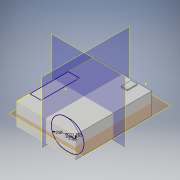
# Autodesk Inventor part: TAZ 6 Convex Model
Saved by Autodesk Inventor 2019 (Build 230136000, 136)
## iProperties
Created: 2021-02-10
Part Number: TAZ 6 Convex Model
Material: Generic
Document SubType Name: Modeling
Designer: Eric
Density: 1 g/cm^3
Appearance: Default
Author: Eric
Autodesk Inventor part; units mm, degrees
ref_plane "YZ Plane" through (0, 0, 0) normal (1, 0, 0) x (0, 1, 0)
ref_plane "XZ Plane" through (0, 0, 0) normal (0, 1, 0) x (-1, 0, 0)
ref_plane "XY Plane" through (0, 0, 0) normal (0, 0, 1) x (1, 0, 0)
ref_plane "Work Plane1" through (-416.1869, -470.7505, 28.2071) normal (0, 0, -1) x (0, 1, 0)
sketch "Sketch1" plane through (-416.1869, -470.7505, 28.2071) normal (0, 0, -1) x (0, 1, 0)
  line L0 (-5.675, 491.5) -> (-5.675, 423.5) construction
  line L1 (170.675, 423.5) -> (170.675, 491.5) construction
  line L2 (166, -7.5) -> (160.638, -7.5) construction
  line L3 (154.362, -7.5) -> (149, -7.5) construction
  line L4 (16, -7.5) -> (10.638, -7.5) construction
  line L5 (4.362, -7.5) -> (-1, -7.5) construction
  line L6 (94.0505, 496.5) -> (100.0959, 496.5) construction
  line L7 (101.0959, 496.5) -> (107.1414, 496.5) construction
  line L8 (108.1414, 496.5) -> (114.1868, 496.5) construction
  line L9 (-13.9999, 496.5) -> (170.675, 496.5)
  line L10 (170.675, 496.5) -> (170.675, -7.5)
  line L11 (170.675, -7.5) -> (-13.9999, -7.5)
  line L12 (-13.9999, -7.5) -> (-13.9999, 496.5)
  line L13 (-13.69, 71.5) -> (-13.69, 253.5) construction
  line L14 (-13.9999, 266.9308) -> (-13.9999, 290.6308) construction
  point P0 (470.7505, 416.1869)
  constraints: 12 end point, 4 collinear, 2 vertical, 4 other
ref_plane "Work Plane2" through (60.3131, -476.4255, 684.8371) normal (0, 0, 1) x (1, 0, 0)
extrude "Extrusion1" add sketch "Sketch1" against normal up to surface (656.63 mm away)
sketch "Sketch2" plane through (-423.6869, -300.0755, 28.2071) normal (0, 1, 0) x (1, 0, 0)
  line L0 (397.25, -16.28) -> (344.1479, -16.28)
  line L1 (344.1479, -16.28) -> (344.1479, -101.13)
  line L2 (344.1479, -101.13) -> (397.25, -101.13)
  line L3 (397.25, -101.13) -> (397.25, -16.28)
  line L4 (344.1479, -35.88) -> (344.1479, -16.38) projected
  arc A0 (397.2117, -88.1724) -> (397.052, -86.959) centre (385.25, -89.13) ccw projected
  line L5 (343.1, -16.28) -> (368.3, -16.28) projected
  point P0 (423.6869, 28.2071)
  constraints: 8 end point, 2 collinear, 2 horizontal, 2 tangent, 2 vertical
ref_plane "Work Plane3" through (-49.4369, -292.7505, 106.3371) normal (0, 1, 0) x (0, 0, 1)
extrude "Extrusion2" add sketch "Sketch2" along normal up to surface (7.325 mm away) separate body
ref_plane "Work Plane4" through (50.3442, -329.0906, 827.6498) normal (0, 0, 1) x (1, 0, 0)
sketch "Sketch4" plane through (-423.6869, -484.7505, 684.8371) normal (0, 0, 1) x (1, 0, 0)
  line L0 (484, 161.1598) -> (484, 161.1598) projected
  line L1 (484, 153.6598) -> (484, 153.6598) projected
  line L2 (504, 157.4099) -> (478, 157.4099)
  line L3 (504, 184.6749) -> (504, 157.4099)
  line L4 (504, 0) -> (0, 0) construction
  line L5 (504, 184.6749) -> (504, 0) construction
  line L6 (0, 184.6749) -> (504, 184.6749) construction
  line L7 (0, 0) -> (0, 184.6749) construction
  line L8 (478, 157.4099) -> (453, 157.4099)
  line L9 (453, 157.4099) -> (423, 157.4099) construction
  line L10 (453, 282.4099) -> (423, 282.4099)
  line L11 (423, 32.4099) -> (453, 32.4099)
  arc A0 (453, 32.4099) -> (453, 282.4099) centre (453, 157.4099) ccw
  arc A1 (423, 282.4099) -> (423, 32.4099) centre (423, 157.4099) ccw
  point P0 (423.6869, 484.7505)
  point P1 (438, 157.4099)
  dimension "d5" = 27.265
  dimension "d6" = 26
  dimension "d7" = 25
  dimension "d9" = 30
  dimension "d10" = 250
  constraints: 14 end point, 4 point on circle, 4 tangent, 3 collinear, 2 centre point, 1 midpoint, 1 parallel, 1 perpendicular
  measures "d5" distance of L3.start L2.start
  measures "d6" distance of L2.start L2.end
  measures "d7" distance of L2.end L8.end
  measures "d9" distance of L8.end L9.end
  measures "d10" diameter of A1
sketch "Sketch6" plane through (-423.6869, -300.0755, 28.2071) normal (0, 1, 0) x (1, 0, 0)
  line L0 (0, 0) -> (0, -656.63) projected
  line L1 (96.005, -527.63) -> (96.005, -227.63) projected
  line L2 (85.43, -212.63) -> (82.255, -212.63) projected
  line L3 (97.505, -212.63) -> (97.505, -234.63) projected
  line L4 (85.43, -212.63) -> (90.255, -212.63) projected
  line L5 (97.505, -520.63) -> (97.505, -542.63) projected
  line L6 (82.255, -542.63) -> (85.43, -542.63) projected
  line L7 (96.005, -212.63) -> (0, -212.63)
  line L8 (0, -212.63) -> (0, -542.63)
  line L9 (0, -542.63) -> (96.005, -542.63)
  line L10 (96.005, -542.63) -> (96.005, -212.63)
  line L11 (96.005, -212.63) -> (99.2801, -212.63) construction
  line L12 (85.43, -542.63) -> (97.505, -542.63)
  point P0 (423.6869, 28.2071)
  constraints: 12 end point, 4 collinear, 3 perpendicular, 1 point on line
ref_plane "Work Plane14" through (-416.1869, -470.7505, 356.5221) normal (0, 0, -1) x (-1, 0, 0)
ref_plane "Work Plane15" through (-171.6869, -484.7505, 28.2071) normal (-1, 0, 0) x (0, 0, 1)
ref_plane "Work Plane17" through (-79.539, -388.7505, 44.4871) normal (0, 1, 0) x (1, 0, 0)
body "Solid1"
body "Solid2"
